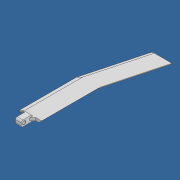
# Autodesk Inventor part: Gyrocopter Blade
Saved by Autodesk Inventor 2022 (Build 260153000, 153)
## iProperties
Created: 2021-12-01
Part Number: Gyrocopter Blade
Material: Generic
Document SubType Name: Modeling
Designer: Vedic
Density: 1 g/cm^3
Appearance: Default
Author: Vedic
Autodesk Inventor part; units mm, degrees
ref_plane "YZ Plane" through (0, 0, 0) normal (1, 0, 0) x (0, 1, 0)
sketch "Sketch1" plane through (0, 0, 0) normal (0, 1, 0) x (-1, 0, 0)
  line L0 (27.5907, 45.377) -> (17.5907, 45.377)
  line L1 (17.5907, 45.377) -> (17.5907, 25.377)
  line L2 (17.5907, 25.377) -> (27.5907, 25.377)
  line L3 (27.5907, 25.377) -> (27.5907, 45.377)
  dimension "d0" = 10
  dimension "d1" = 20
  constraints: 8 end point, 2 parallel, 1 horizontal, 1 perpendicular
  measures "d0" distance of L0.start L0.end
  measures "d1" distance of L2.end L0.start
extrude "Extrusion1" add sketch "Sketch1" along normal blind 10
sketch "Sketch2" plane through (-17.5907, 0, 45.377) normal (1, 0, 0) x (0, 0, -1)
  line L0 (0, 10) -> (20, 10) construction
  line L1 (0, 10) -> (10, 10) construction
  line L2 (10, 10) -> (10, 0) construction
  line L3 (10, 0) -> (0, 0) construction
  line L4 (0, 0) -> (0, 10) construction
  line L5 (20, 0) -> (20, 10) construction
  line L6 (0, 10) -> (10, 0) construction
  line L7 (0, 0) -> (20, 0) construction
  line L8 (10, 10) -> (0, 0) construction
  circle A0 centre (5, 5) radius 2.5
  point P0 (45.377, 0)
  dimension "d4" = 5
  constraints: 12 end point, 2 equal length, 2 parallel, 2 perpendicular, 1 centre point, 1 horizontal, 1 midpoint
  measures "d4" diameter of A0
extrude "Extrusion2" cut sketch "Sketch2" against normal through all
fillet "Fillet1" radius 0.5 2 edges at (-17.5907, 5, 42.877) (-27.5907, 5, 42.877)
fillet "Fillet2" radius 3 2 edges at (-22.5907, 10, 45.377) (-22.5907, 0, 45.377)
ref_plane "Work Plane1" through (0, 7.5, 0) normal (0, 1, 0) x (1, 0, 0)
ref_plane "Work Plane2" through (0, 2.5, 0) normal (0, -1, 0) x (1, 0, 0)
sketch "Sketch7" plane through (0, 7.5, 0) normal (0, 1, 0) x (1, 0, 0)
  line L0 (-32.5907, -25.377) -> (-2.5907, -25.377)
  line L1 (-2.5907, -25.377) -> (-2.5907, 74.623)
  line L2 (-2.5907, 74.623) -> (-32.5907, 74.623)
  line L3 (-32.5907, 74.623) -> (-32.5907, -25.377)
  line L4 (-17.5907, -25.377) -> (-27.5907, -25.377) projected
  line L5 (-27.5907, -25.377) -> (-27.5907, -42.377) projected
  line L6 (-17.5907, -42.377) -> (-17.5907, -25.377) projected
  point P0 (0, 0)
  dimension "d30" = 0
  dimension "d31" = 5
  dimension "d32" = 15
  dimension "d33" = 100
  constraints: 8 end point, 2 parallel, 1 horizontal, 1 perpendicular
  measures "d30" distance between parallel lines of L4 L0
  measures "d31" distance between parallel lines of L3 L5
  measures "d32" distance from line of L0.end L6
  measures "d33" distance of L2.end L0.start
sketch "Sketch8" plane through (0, 2.5, 0) normal (0, -1, 0) x (1, 0, 0)
  line L0 (-42.5907, 25.377) -> (-7.5907, 25.377)
  line L1 (-7.5907, 25.377) -> (-7.5907, -74.623)
  line L2 (-7.5907, -74.623) -> (-42.5907, -74.623)
  line L3 (-42.5907, -74.623) -> (-42.5907, 25.377)
  line L4 (-17.5907, 25.377) -> (-27.5907, 25.377) projected
  line L5 (-27.5907, 25.377) -> (-27.5907, 42.377) projected
  line L6 (-17.5907, 42.377) -> (-17.5907, 25.377) projected
  point P0 (0, 0)
  dimension "d34" = 0
  dimension "d35" = 15
  dimension "d36" = 10
  dimension "d37" = 100
  constraints: 8 end point, 2 parallel, 1 horizontal, 1 perpendicular
  measures "d34" distance between parallel lines of L4 L0
  measures "d35" distance between parallel lines of L5 L3
  measures "d36" distance between parallel lines of L6 L1
  measures "d37" distance of L2.end L0.start
loft "Loft4" add profiles "Sketch8", "Sketch7"
sketch "Sketch9" plane through (-17.5907, 0, 42.377) normal (1, 0, 0) x (0, 0, -1)
  line L0 (17, 7.5) -> (17, 10) projected
  line L1 (17, 7.5) -> (12, 7.5)
  line L2 (12, 7.5) -> (12, 2.5)
  line L3 (12, 2.5) -> (17, 2.5)
  line L4 (17, 2.5) -> (17, 7.5)
  line L5 (17, 0) -> (17, 2.5) projected
  point P0 (42.377, 0)
  dimension "d42" = 5
  constraints: 8 end point, 2 parallel, 1 horizontal, 1 perpendicular
  measures "d42" distance of L0.start L1.end
sketch "Sketch10" plane through (-27.5907, 0, 25.377) normal (-1, 0, 0) x (0, 0, 1)
  line L0 (0, 2.5) -> (0, 7.5) projected
  line L1 (0, 7.5) -> (5, 7.5)
  line L2 (5, 7.5) -> (5, 2.5)
  line L3 (5, 2.5) -> (0, 2.5)
  line L4 (0, 2.5) -> (0, 7.5)
  point P0 (-25.377, 0)
  dimension "d43" = 5
  constraints: 8 end point, 2 parallel, 1 horizontal, 1 perpendicular
  measures "d43" distance of L2.end L0.start
extrude "Extrusion3" add sketch "Sketch10" along normal blind 5
extrude "Extrusion4" add sketch "Sketch9" along normal blind 5
chamfer "Chamfer1" distance 5 angle 45 2 edges at (-12.5907, 5, 30.377) (-32.5907, 5, 30.377)
sketch "Sketch11" plane through (-32.5907, 7.5, -74.623) normal (0, 1, 0) x (1, 0, 0)
  line L0 (30, 0) -> (0, 0) projected
  line L1 (30, 0) -> (56.7949, 100)
  line L2 (56.7949, 100) -> (26.7949, 100)
  line L3 (26.7949, 100) -> (0, 0)
  line L4 (30, -100) -> (30, 0) projected
  point P0 (32.5907, -74.623)
  dimension "d52" = 15
  dimension "d53" = 100
  constraints: 6 end point, 2 parallel
  measures "d52" angle of L1 L4
  measures "d53" distance between parallel lines of L0 L2
sketch "Sketch12" plane through (-42.5907, 2.5, -74.623) normal (0, -1, 0) x (1, 0, 0)
  line L0 (35, 0) -> (0, 0) projected
  line L1 (0, 0) -> (26.7949, -100)
  line L2 (26.7949, -100) -> (61.7949, -100)
  line L3 (61.7949, -100) -> (35, 0)
  line L4 (0, 0) -> (0, 100) projected
  point P0 (42.5907, 74.623)
  dimension "d54" = 100
  dimension "d55" = 15
  constraints: 6 end point, 2 parallel
  measures "d54" distance between parallel lines of L2 L0
  measures "d55" angle of L1 L4
loft "Loft5" add profiles "Sketch11", "Sketch12"
chamfer "Chamfer2" distance 2.5 angle 45 2 edges at (-22.5907, 0, 25.377) (-22.5907, 10, 25.377)
chamfer "Chamfer3" distance 2.5 angle 45 1 edges at (9.2042, 7.5, -174.623)
equation "\"d35\" = d32"
equation "\"d37\" = d33"
equation "\"d43\" = d42"
equation "\"d54\" = d53"
equation "\"d55\" = d52"
body "Solid1"
